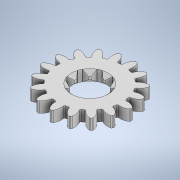
# Autodesk Inventor part: Gear_input
Saved by Autodesk Inventor 2020 (Build 240168000, 168)
## iProperties
Created: 2020-05-11
Part Number: Gear_input
Material: Generic
Document SubType Name: Modeling
Designer: avi41
Density: 1 g/cm^3
Appearance: Default
Author: avi41
Autodesk Inventor part; units mm, degrees
ref_plane "YZ Plane" through (0, 0, 0) normal (1, 0, 0) x (0, 1, 0)
ref_plane "XZ Plane" through (0, 0, 0) normal (0, 1, 0) x (-1, 0, 0)
ref_plane "XY Plane" through (0, 0, 0) normal (0, 0, 1) x (1, 0, 0)
sketch "Sketch1" plane through (0, 0, 0) normal (0, 1, 0) x (-1, 0, 0)
  arc A0 (0.3488, -8.9491) -> (-2.2796, -8.6609) centre (0, 0) ccw construction
  line L0 (0, -21.7523) -> (0, 17.3166) construction
  line L1 (-16.4294, 0) -> (16.4294, 0) construction
  arc A1 (0.3488, -8.9491) -> (-2.2796, -8.6609) centre (0, 0) ccw
  circle A2 centre (0, 0) radius 11.7353 construction
  circle A3 centre (0, 0) radius 10.5 construction
  line L2 (0, 0) -> (-4.0137, -11.0276) construction
  circle A4 centre (0, 0) radius 9.8668 construction
  line L3 (-3.3746, -9.2717) -> (5.3254, -12.4383) construction
  line L4 (3.5046, -9.8668) -> (-4.0266, -9.8668) construction
  arc A5 (-0.9533, -11.6965) -> (0.052, -9.2588) centre (-3.3746, -9.2717) ccw
  circle A6 centre (0, 0) radius 9.2647 construction
  arc A7 (0.3488, -8.9491) -> (0.052, -9.2588) centre (0.3609, -9.2577) ccw
  line L5 (-1.3339, -12.1661) -> (-0.7958, -7.2586) construction
  arc A8 (-2.057, -9.0276) -> (-1.6037, -11.6252) centre (1.2855, -9.7827) ccw
  arc A9 (-2.057, -9.0276) -> (-2.2796, -8.6609) centre (-2.3582, -8.9595) ccw
  line L6 (-0.9533, -11.6965) -> (-1.6037, -11.6252)
  point P0 (0, -9.8668)
  point P1 (-0.149, -9.2635)
  point P2 (0, -16.1711)
  point P3 (-0.1751, -10.4985)
  point P4 (-1.8617, -9.0757)
  point P5 (-3.504, -15.7869)
  point P6 (-0.1601, -15.8391)
  point P7 (-6.1857, -13.0529)
  point P8 (-5.7886, -14.7444)
  point P9 (-1.2807, -6.5842)
  dimension "d23" = 21
  dimension "d25" = 1.5441
  dimension "d26" = 1.2353
  dimension "d27" = 20
  dimension "d28" = 19.7336
  dimension "d29" = 20
  dimension "d30" = 0.3088
  dimension "d31" = 0.6177
  dimension "d32" = 0.9702
  constraints: 18 point on circle, 10 end point, 8 centre point, 7 coincident, 6 symmetric about line, 4 point on line, 3 tangent, 1 concentric, 1 horizontal, 8 other
  measures "d27" angle of L0 L2
  measures "d28" diameter of A4
  measures "d29" angle of L4 L3
  measures "d31" diameter of A7
  measures "d32" distance from line of point (-0.175, -10.499) L5
extrude "Extrusion1" add sketch "Sketch1" along normal mid plane 3
fillet "Fillet2" radius 0.4 2 edges at (0.9533, 0, -11.6965) (1.6037, 0, -11.6252)
pattern_circular "Circular Pattern2" count 17 over 360 about axis through (0, -10, 0) along (0, 1, 0) of "Extrusion1", "Fillet2"
sketch "Sketch3" plane through (0, 0, 0) normal (0, 1, 0) x (-1, 0, 0)
  line L0 (-7, 0) -> (7, 0) construction
  line L1 (0, 7) -> (0, -7) construction
  circle A0 centre (0, 0) radius 4.9 construction
  circle A1 centre (0, 0) radius 3.8 construction
  line L2 (-0.5, 4.8744) -> (-1.2405, 3.5918) construction
  line L3 (0.5, 4.8744) -> (1.2405, 3.5918) construction
  circle A2 centre (0, 0) radius 3.75 construction
  circle A3 centre (0, 0) radius 4.45 construction
  circle A4 centre (-1.3496, 3.7229) radius 0.16 construction
  circle A5 centre (1.3496, 3.7229) radius 0.16 construction
  circle A6 centre (0, 0) radius 3.8 construction
  line L4 (0.5, 4.8744) -> (1.2405, 3.5918) construction
  line L5 (-0.5, 4.8744) -> (-1.2405, 3.5918) construction
  arc A7 (-1.2951, 3.5725) -> (-1.211, 3.6429) centre (-1.3496, 3.7229) ccw construction
  arc A8 (1.211, 3.6429) -> (1.2951, 3.5725) centre (1.3496, 3.7229) ccw construction
  arc A9 (0.5, 4.8744) -> (-0.5, 4.8744) centre (0, 0) ccw construction
  circle A10 centre (0, 0) radius 3.8 construction
  circle A11 centre (0, 0) radius 3.8 construction
  circle A12 centre (0, 0) radius 4.45 construction
  circle A13 centre (0, 0) radius 3.75 construction
  circle A14 centre (0, 0) radius 4.9 construction
  arc A15 (-1.7196, 3.4323) -> (-1.6104, 3.4419) centre (-1.6782, 3.5868) ccw construction
  circle A16 centre (-1.6782, 3.5868) radius 0.16 construction
  arc A17 (-3.0932, 3.8003) -> (-3.8003, 3.0932) centre (0, 0) ccw construction
  line L6 (-3.0932, 3.8003) -> (-1.6626, 3.417) construction
  line L7 (-3.0932, 3.8003) -> (-1.6626, 3.417) construction
  line L8 (-3.8003, 3.0932) -> (-3.417, 1.6626) construction
  line L9 (-3.8003, 3.0932) -> (-3.417, 1.6626) construction
  arc A18 (-3.4419, 1.6104) -> (-3.4323, 1.7196) centre (-3.5868, 1.6782) ccw construction
  circle A19 centre (-3.5868, 1.6782) radius 0.16 construction
  circle A20 centre (0, 0) radius 3.8 construction
  circle A21 centre (0, 0) radius 3.8 construction
  circle A22 centre (0, 0) radius 4.45 construction
  circle A23 centre (0, 0) radius 3.75 construction
  circle A24 centre (0, 0) radius 4.9 construction
  arc A25 (-3.6429, 1.211) -> (-3.5725, 1.2951) centre (-3.7229, 1.3496) ccw construction
  circle A26 centre (-3.7229, 1.3496) radius 0.16 construction
  arc A27 (-4.8744, 0.5) -> (-4.8744, -0.5) centre (0, 0) ccw construction
  line L10 (-4.8744, 0.5) -> (-3.5918, 1.2405) construction
  line L11 (-4.8744, 0.5) -> (-3.5918, 1.2405) construction
  line L12 (-4.8744, -0.5) -> (-3.5918, -1.2405) construction
  line L13 (-4.8744, -0.5) -> (-3.5918, -1.2405) construction
  arc A28 (-3.5725, -1.2951) -> (-3.6429, -1.211) centre (-3.7229, -1.3496) ccw construction
  circle A29 centre (-3.7229, -1.3496) radius 0.16 construction
  circle A30 centre (0, 0) radius 3.8 construction
  circle A31 centre (0, 0) radius 3.8 construction
  circle A32 centre (0, 0) radius 4.45 construction
  circle A33 centre (0, 0) radius 3.75 construction
  circle A34 centre (0, 0) radius 4.9 construction
  arc A35 (-3.4323, -1.7196) -> (-3.4419, -1.6104) centre (-3.5868, -1.6782) ccw construction
  circle A36 centre (-3.5868, -1.6782) radius 0.16 construction
  arc A37 (-3.8003, -3.0932) -> (-3.0932, -3.8003) centre (0, 0) ccw construction
  line L14 (-3.8003, -3.0932) -> (-3.417, -1.6626) construction
  line L15 (-3.8003, -3.0932) -> (-3.417, -1.6626) construction
  line L16 (-3.0932, -3.8003) -> (-1.6626, -3.417) construction
  line L17 (-3.0932, -3.8003) -> (-1.6626, -3.417) construction
  arc A38 (-1.6104, -3.4419) -> (-1.7196, -3.4323) centre (-1.6782, -3.5868) ccw construction
  circle A39 centre (-1.6782, -3.5868) radius 0.16 construction
  circle A40 centre (0, 0) radius 3.8 construction
  circle A41 centre (0, 0) radius 3.8 construction
  circle A42 centre (0, 0) radius 4.45 construction
  circle A43 centre (0, 0) radius 3.75 construction
  circle A44 centre (0, 0) radius 4.9 construction
  arc A45 (-1.211, -3.6429) -> (-1.2951, -3.5725) centre (-1.3496, -3.7229) ccw construction
  circle A46 centre (-1.3496, -3.7229) radius 0.16 construction
  arc A47 (-0.5, -4.8744) -> (0.5, -4.8744) centre (0, 0) ccw construction
  line L18 (-0.5, -4.8744) -> (-1.2405, -3.5918) construction
  line L19 (-0.5, -4.8744) -> (-1.2405, -3.5918) construction
  line L20 (0.5, -4.8744) -> (1.2405, -3.5918) construction
  line L21 (0.5, -4.8744) -> (1.2405, -3.5918) construction
  arc A48 (1.2951, -3.5725) -> (1.211, -3.6429) centre (1.3496, -3.7229) ccw construction
  circle A49 centre (1.3496, -3.7229) radius 0.16 construction
  circle A50 centre (0, 0) radius 3.8 construction
  circle A51 centre (0, 0) radius 3.8 construction
  circle A52 centre (0, 0) radius 4.45 construction
  circle A53 centre (0, 0) radius 3.75 construction
  circle A54 centre (0, 0) radius 4.9 construction
  arc A55 (1.7196, -3.4323) -> (1.6104, -3.4419) centre (1.6782, -3.5868) ccw construction
  circle A56 centre (1.6782, -3.5868) radius 0.16 construction
  arc A57 (3.0932, -3.8003) -> (3.8003, -3.0932) centre (0, 0) ccw construction
  line L22 (3.0932, -3.8003) -> (1.6626, -3.417) construction
  line L23 (3.0932, -3.8003) -> (1.6626, -3.417) construction
  line L24 (3.8003, -3.0932) -> (3.417, -1.6626) construction
  line L25 (3.8003, -3.0932) -> (3.417, -1.6626) construction
  arc A58 (3.4419, -1.6104) -> (3.4323, -1.7196) centre (3.5868, -1.6782) ccw construction
  circle A59 centre (3.5868, -1.6782) radius 0.16 construction
  circle A60 centre (0, 0) radius 3.8 construction
  circle A61 centre (0, 0) radius 3.8 construction
  circle A62 centre (0, 0) radius 4.45 construction
  circle A63 centre (0, 0) radius 3.75 construction
  circle A64 centre (0, 0) radius 4.9 construction
  arc A65 (3.6429, -1.211) -> (3.5725, -1.2951) centre (3.7229, -1.3496) ccw construction
  circle A66 centre (3.7229, -1.3496) radius 0.16 construction
  arc A67 (4.8744, -0.5) -> (4.8744, 0.5) centre (0, 0) ccw construction
  line L26 (4.8744, -0.5) -> (3.5918, -1.2405) construction
  line L27 (4.8744, -0.5) -> (3.5918, -1.2405) construction
  line L28 (4.8744, 0.5) -> (3.5918, 1.2405) construction
  line L29 (4.8744, 0.5) -> (3.5918, 1.2405) construction
  arc A68 (3.5725, 1.2951) -> (3.6429, 1.211) centre (3.7229, 1.3496) ccw construction
  circle A69 centre (3.7229, 1.3496) radius 0.16 construction
  line L30 (0, -16.3542) -> (0, 16.3851) construction
  line L31 (-16.3961, 0) -> (16.2574, 0) construction
  circle A70 centre (0, 0) radius 4
  circle A71 centre (0, 0) radius 5.1 construction
  line L32 (1.4495, 4.8897) -> (0.2774, 3.9904) construction
  line L33 (-1.4495, 4.8897) -> (-0.2774, 3.9904) construction
  arc A72 (-1.3841, 4.8395) -> (-1.5295, 4.8652) centre (-1.4815, 4.7126) ccw
  arc A73 (1.5295, 4.8652) -> (1.3841, 4.8395) centre (1.4815, 4.7126) ccw
  line L34 (1.3841, 4.8395) -> (0.2774, 3.9904)
  line L35 (-1.3841, 4.8395) -> (-0.2774, 3.9904)
  circle A74 centre (0, 0) radius 5.1
  circle A75 centre (0, 0) radius 4.45 construction
  line L36 (-4.4825, 2.4326) -> (-3.0178, 2.6254) construction
  arc A76 (-4.4008, 2.4434) -> (-4.5218, 2.3587) centre (-4.3799, 2.2847) ccw
  line L37 (-2.4434, 4.4008) -> (-2.6254, 3.0178)
  arc A77 (-2.3587, 4.5218) -> (-2.4434, 4.4008) centre (-2.2847, 4.3799) ccw
  line L38 (-2.4326, 4.4825) -> (-2.6254, 3.0178) construction
  line L39 (-4.4008, 2.4434) -> (-3.0178, 2.6254)
  line L40 (-4.8897, -1.4495) -> (-3.9904, -0.2774) construction
  arc A78 (-4.8395, -1.3841) -> (-4.8652, -1.5295) centre (-4.7126, -1.4815) ccw
  line L41 (-4.8395, 1.3841) -> (-3.9904, 0.2774)
  arc A79 (-4.8652, 1.5295) -> (-4.8395, 1.3841) centre (-4.7126, 1.4815) ccw
  line L42 (-4.8897, 1.4495) -> (-3.9904, 0.2774) construction
  line L43 (-4.8395, -1.3841) -> (-3.9904, -0.2774)
  line L44 (-2.4326, -4.4825) -> (-2.6254, -3.0178) construction
  arc A80 (-2.4434, -4.4008) -> (-2.3587, -4.5218) centre (-2.2847, -4.3799) ccw
  line L45 (-4.4008, -2.4434) -> (-3.0178, -2.6254)
  arc A81 (-4.5218, -2.3587) -> (-4.4008, -2.4434) centre (-4.3799, -2.2847) ccw
  line L46 (-4.4825, -2.4326) -> (-3.0178, -2.6254) construction
  line L47 (-2.4434, -4.4008) -> (-2.6254, -3.0178)
  line L48 (1.4495, -4.8897) -> (0.2774, -3.9904) construction
  arc A82 (1.3841, -4.8395) -> (1.5295, -4.8652) centre (1.4815, -4.7126) ccw
  line L49 (-1.3841, -4.8395) -> (-0.2774, -3.9904)
  arc A83 (-1.5295, -4.8652) -> (-1.3841, -4.8395) centre (-1.4815, -4.7126) ccw
  line L50 (-1.4495, -4.8897) -> (-0.2774, -3.9904) construction
  line L51 (1.3841, -4.8395) -> (0.2774, -3.9904)
  line L52 (4.4825, -2.4326) -> (3.0178, -2.6254) construction
  arc A84 (4.4008, -2.4434) -> (4.5218, -2.3587) centre (4.3799, -2.2847) ccw
  line L53 (2.4434, -4.4008) -> (2.6254, -3.0178)
  arc A85 (2.3587, -4.5218) -> (2.4434, -4.4008) centre (2.2847, -4.3799) ccw
  line L54 (2.4326, -4.4825) -> (2.6254, -3.0178) construction
  line L55 (4.4008, -2.4434) -> (3.0178, -2.6254)
  line L56 (4.8897, 1.4495) -> (3.9904, 0.2774) construction
  arc A86 (4.8395, 1.3841) -> (4.8652, 1.5295) centre (4.7126, 1.4815) ccw
  line L57 (4.8395, -1.3841) -> (3.9904, -0.2774)
  arc A87 (4.8652, -1.5295) -> (4.8395, -1.3841) centre (4.7126, -1.4815) ccw
  line L58 (4.8897, -1.4495) -> (3.9904, -0.2774) construction
  line L59 (4.8395, 1.3841) -> (3.9904, 0.2774)
  circle A88 centre (0, 0) radius 3.8 construction
  circle A89 centre (0, 0) radius 3.8 construction
  circle A90 centre (0, 0) radius 4.45 construction
  circle A91 centre (0, 0) radius 3.75 construction
  circle A92 centre (0, 0) radius 4.9 construction
  arc A93 (3.4323, 1.7196) -> (3.4419, 1.6104) centre (3.5868, 1.6782) ccw construction
  circle A94 centre (3.5868, 1.6782) radius 0.16 construction
  arc A95 (3.8003, 3.0932) -> (3.0932, 3.8003) centre (0, 0) ccw construction
  line L60 (3.8003, 3.0932) -> (3.417, 1.6626) construction
  line L61 (3.8003, 3.0932) -> (3.417, 1.6626) construction
  line L62 (3.0932, 3.8003) -> (1.6626, 3.417) construction
  line L63 (3.0932, 3.8003) -> (1.6626, 3.417) construction
  arc A96 (1.6104, 3.4419) -> (1.7196, 3.4323) centre (1.6782, 3.5868) ccw construction
  circle A97 centre (1.6782, 3.5868) radius 0.16 construction
  line L64 (2.4326, 4.4825) -> (2.6254, 3.0178) construction
  arc A98 (2.4434, 4.4008) -> (2.3587, 4.5218) centre (2.2847, 4.3799) ccw
  line L65 (4.4008, 2.4434) -> (3.0178, 2.6254)
  arc A99 (4.5218, 2.3587) -> (4.4008, 2.4434) centre (4.3799, 2.2847) ccw
  line L66 (4.4825, 2.4326) -> (3.0178, 2.6254) construction
  line L67 (2.4434, 4.4008) -> (2.6254, 3.0178)
  point P0 (-0.7854, 4.3801)
  point P1 (0.7854, 4.3801)
  point P2 (-3.6526, 2.5419)
  point P3 (-2.5419, 3.6526)
  point P4 (-4.3801, -0.7854)
  point P5 (-4.3801, 0.7854)
  point P6 (-2.5419, -3.6526)
  point P7 (-3.6526, -2.5419)
  point P8 (0.7854, -4.3801)
  point P9 (-0.7854, -4.3801)
  point P10 (3.6526, -2.5419)
  point P11 (2.5419, -3.6526)
  point P12 (4.3801, 0.7854)
  point P13 (4.3801, -0.7854)
  point P14 (1.3297, 2.7449)
  point P15 (2.9719, 0.6856)
  point P16 (2.9751, 0.6718)
  point P17 (2.389, -1.8961)
  point P18 (2.3802, -1.9072)
  point P19 (0.0071, -3.05)
  point P20 (-0.0071, -3.05)
  point P21 (-2.3802, -1.9072)
  point P22 (-2.389, -1.8961)
  point P23 (-2.9751, 0.6718)
  point P24 (-2.9719, 0.6856)
  point P25 (-1.3297, 2.7449)
  point P26 (0.7854, 4.3801)
  point P27 (-0.7854, 4.3801)
  point P28 (-2.5419, 3.6526)
  point P29 (-3.6526, 2.5419)
  point P30 (-4.3801, 0.7854)
  point P31 (-4.3801, -0.7854)
  point P32 (-3.6526, -2.5419)
  point P33 (-2.5419, -3.6526)
  point P34 (-0.7854, -4.3801)
  point P35 (0.7854, -4.3801)
  point P36 (2.5419, -3.6526)
  point P37 (3.6526, -2.5419)
  point P38 (4.3801, -0.7854)
  point P39 (4.3801, 0.7854)
  point P40 (3.9904, 0.2774)
  point P41 (4.8652, 1.5295)
  point P42 (-2.3587, 4.5218)
  point P43 (-2.6254, 3.0178)
  point P44 (-3.0178, 2.6254)
  point P45 (-4.5218, 2.3587)
  point P46 (-4.8652, 1.5295)
  point P47 (-3.9904, 0.2774)
  point P48 (-3.9904, -0.2774)
  point P49 (-4.8652, -1.5295)
  point P50 (-4.5218, -2.3587)
  point P51 (-3.0178, -2.6254)
  point P52 (-2.6254, -3.0178)
  point P53 (-2.3587, -4.5218)
  point P54 (-1.5295, -4.8652)
  point P55 (-0.2774, -3.9904)
  point P56 (0.2774, -3.9904)
  point P57 (1.5295, -4.8652)
  point P58 (2.3587, -4.5218)
  point P59 (2.6254, -3.0178)
  point P60 (3.0178, -2.6254)
  point P61 (4.5218, -2.3587)
  point P62 (4.8652, -1.5295)
  point P63 (3.9904, -0.2774)
  point P64 (2.5419, 3.6526)
  point P65 (3.6526, 2.5419)
  point P66 (3.6526, 2.5419)
  point P67 (2.5419, 3.6526)
  point P68 (2.6254, 3.0178)
  point P69 (2.3587, 4.5218)
  point P70 (4.5218, 2.3587)
  point P71 (3.0178, 2.6254)
  dimension "d36" = 9.8
  dimension "d37" = 7.6
  dimension "d38" = 30
  dimension "d39" = 7.5
  dimension "d40" = 0.65
  dimension "d41" = 1.5708
  dimension "d42" = 0.32
  dimension "d43" = 360
  dimension "d58" = 8
  dimension "d59" = 10.2
  dimension "d60" = 8.9
  dimension "d61" = 1.5708
  dimension "d68" = 360
  dimension "d74" = 60
  constraints: 152 point on circle, 132 end point, 100 centre point, 64 point on line, 61 coincident, 8 tangent, 6 equal radius, 3 collinear, 3 midpoint, 2 horizontal, 2 vertical, 1 symmetric about line, 465 other
  measures "d36" diameter of A0
  measures "d37" diameter of A1
  measures "d38" angle of L1 L2
  measures "d39" diameter of A2
  measures "d40" radial gap between concentric circles of A3 A1
  measures "d41" distance of A3.end A3.start
  measures "d42" diameter of A4
  measures "d58" diameter of A70
  measures "d59" diameter of A71
  measures "d60" diameter of A75
  measures "d61" distance of A75.start A75.end
  measures "d74" angle of L64 L34
extrude "Extrusion4" cut sketch "Sketch3" against normal through all both and the other way through all contours A70 | A70 L65 A99 A74 A86 L59 | L57 A87 A74 A84 L55 A70 | A70 L34 A73 A74 A98 L67 | L53 A85 A74 A82 L51 A70 | A70 L37 A77 A74 A72 L35 | L49 A83 A74 A80 L47 A70 | A70 L41 A79 A74 A76 L39 | L45 A81 A74 A78 L43 A70
sketch "Sketch4" plane through (0, 1.5, 0) normal (0, 1, 0) x (1, 0, 0)
  circle A0 centre (0, 0) radius 5.1
  arc A1 (-2.4434, -4.4008) -> (-2.3587, -4.5218) centre (-2.2847, -4.3799) ccw projected
  line L0 (-2.4434, -4.4008) -> (-2.6254, -3.0178) projected
  arc A2 (-3.0178, -2.6254) -> (-2.6254, -3.0178) centre (0, 0) ccw projected
  line L1 (-3.0178, -2.6254) -> (-4.4008, -2.4434) projected
  arc A3 (-4.5218, -2.3587) -> (-4.4008, -2.4434) centre (-4.3799, -2.2847) ccw projected
  arc A4 (-4.8652, -1.5295) -> (-4.5218, -2.3587) centre (0, 0) ccw projected
  arc A5 (-4.8395, -1.3841) -> (-4.8652, -1.5295) centre (-4.7126, -1.4815) ccw projected
  line L2 (-4.8395, -1.3841) -> (-3.9904, -0.2774) projected
  arc A6 (-3.9904, 0.2774) -> (-3.9904, -0.2774) centre (0, 0) ccw projected
  line L3 (-3.9904, 0.2774) -> (-4.8395, 1.3841) projected
  arc A7 (-4.8652, 1.5295) -> (-4.8395, 1.3841) centre (-4.7126, 1.4815) ccw projected
  arc A8 (-4.5218, 2.3587) -> (-4.8652, 1.5295) centre (0, 0) ccw projected
  arc A9 (-4.4008, 2.4434) -> (-4.5218, 2.3587) centre (-4.3799, 2.2847) ccw projected
  line L4 (-4.4008, 2.4434) -> (-3.0178, 2.6254) projected
  arc A10 (-2.6254, 3.0178) -> (-3.0178, 2.6254) centre (0, 0) ccw projected
  line L5 (-2.6254, 3.0178) -> (-2.4434, 4.4008) projected
  arc A11 (-2.3587, 4.5218) -> (-2.4434, 4.4008) centre (-2.2847, 4.3799) ccw projected
  arc A12 (-1.5295, 4.8652) -> (-2.3587, 4.5218) centre (0, 0) ccw projected
  arc A13 (-1.3841, 4.8395) -> (-1.5295, 4.8652) centre (-1.4815, 4.7126) ccw projected
  line L6 (-1.3841, 4.8395) -> (-0.2774, 3.9904) projected
  arc A14 (0.2774, 3.9904) -> (-0.2774, 3.9904) centre (0, 0) ccw projected
  line L7 (0.2774, 3.9904) -> (1.3841, 4.8395) projected
  arc A15 (1.5295, 4.8652) -> (1.3841, 4.8395) centre (1.4815, 4.7126) ccw projected
  arc A16 (2.3587, 4.5218) -> (1.5295, 4.8652) centre (0, 0) ccw projected
  arc A17 (2.4434, 4.4008) -> (2.3587, 4.5218) centre (2.2847, 4.3799) ccw projected
  line L8 (2.4434, 4.4008) -> (2.6254, 3.0178) projected
  arc A18 (3.0178, 2.6254) -> (2.6254, 3.0178) centre (0, 0) ccw projected
  line L9 (3.0178, 2.6254) -> (4.4008, 2.4434) projected
  arc A19 (4.5218, 2.3587) -> (4.4008, 2.4434) centre (4.3799, 2.2847) ccw projected
  arc A20 (4.8652, 1.5295) -> (4.5218, 2.3587) centre (0, 0) ccw projected
  arc A21 (4.8395, 1.3841) -> (4.8652, 1.5295) centre (4.7126, 1.4815) ccw projected
  line L10 (4.8395, 1.3841) -> (3.9904, 0.2774) projected
  arc A22 (3.9904, -0.2774) -> (3.9904, 0.2774) centre (0, 0) ccw projected
  line L11 (3.9904, -0.2774) -> (4.8395, -1.3841) projected
  arc A23 (4.8652, -1.5295) -> (4.8395, -1.3841) centre (4.7126, -1.4815) ccw projected
  arc A24 (4.5218, -2.3587) -> (4.8652, -1.5295) centre (0, 0) ccw projected
  arc A25 (4.4008, -2.4434) -> (4.5218, -2.3587) centre (4.3799, -2.2847) ccw projected
  line L12 (4.4008, -2.4434) -> (3.0178, -2.6254) projected
  arc A26 (2.6254, -3.0178) -> (3.0178, -2.6254) centre (0, 0) ccw projected
  line L13 (2.6254, -3.0178) -> (2.4434, -4.4008) projected
  arc A27 (2.3587, -4.5218) -> (2.4434, -4.4008) centre (2.2847, -4.3799) ccw projected
  arc A28 (1.5295, -4.8652) -> (2.3587, -4.5218) centre (0, 0) ccw projected
  arc A29 (1.3841, -4.8395) -> (1.5295, -4.8652) centre (1.4815, -4.7126) ccw projected
  line L14 (1.3841, -4.8395) -> (0.2774, -3.9904) projected
  arc A30 (-0.2774, -3.9904) -> (0.2774, -3.9904) centre (0, 0) ccw projected
  line L15 (-0.2774, -3.9904) -> (-1.3841, -4.8395) projected
  arc A31 (-1.5295, -4.8652) -> (-1.3841, -4.8395) centre (-1.4815, -4.7126) ccw projected
  arc A32 (-2.3587, -4.5218) -> (-1.5295, -4.8652) centre (0, 0) ccw projected
  arc A33 (2.057, 9.0276) -> (2.2796, 8.6609) centre (2.3582, 8.9595) ccw projected
  arc A34 (2.057, 9.0276) -> (1.7121, 11.4431) centre (-1.2855, 9.7827) ccw projected
  arc A35 (1.7121, 11.4431) -> (1.4058, 11.6469) centre (1.3622, 11.2493) ccw projected
  line L16 (1.4058, 11.6469) -> (1.1513, 11.6748) projected
  arc A36 (1.1513, 11.6748) -> (0.8081, 11.5422) centre (1.1077, 11.2772) ccw projected
  arc A37 (0.8081, 11.5422) -> (-0.052, 9.2588) centre (3.3746, 9.2717) ccw projected
  arc A38 (-0.3488, 8.9491) -> (-0.052, 9.2588) centre (-0.3609, 9.2577) ccw projected
  arc A39 (-0.3488, 8.9491) -> (-1.003, 8.8995) centre (0, 0) ccw projected
  arc A40 (-1.343, 9.1611) -> (-1.003, 8.8995) centre (-1.0376, 9.2064) ccw projected
  arc A41 (-1.343, 9.1611) -> (-2.5373, 11.2889) centre (-4.7326, 8.6577) ccw projected
  arc A42 (-2.5373, 11.2889) -> (-2.8965, 11.3682) centre (-2.7935, 10.9817) ccw projected
  line L17 (-2.8965, 11.3682) -> (-3.1439, 11.3023) projected
  arc A43 (-3.1439, 11.3023) -> (-3.416, 11.0547) centre (-3.0409, 10.9158) ccw projected
  arc A44 (-3.416, 11.0547) -> (-3.3932, 8.6148) centre (-0.2026, 9.8647) ccw projected
  arc A45 (-3.5581, 8.2188) -> (-3.3932, 8.6148) centre (-3.6807, 8.5022) ccw projected
  arc A46 (-3.5581, 8.2188) -> (-4.1501, 7.9363) centre (0, 0) ccw projected
  arc A47 (-4.5617, 8.0573) -> (-4.1501, 7.9363) centre (-4.2932, 8.2099) ccw projected
  arc A48 (-4.5617, 8.0573) -> (-6.4439, 9.61) centre (-7.5405, 6.3635) ccw projected
  arc A49 (-6.4439, 9.61) -> (-6.8076, 9.5542) centre (-6.5719, 9.231) ccw projected
  line L18 (-6.8076, 9.5542) -> (-7.0145, 9.4034) projected
  arc A50 (-7.0145, 9.4034) -> (-7.1788, 9.0742) centre (-6.7788, 9.0802) ccw projected
  arc A51 (-7.1788, 9.0742) -> (-6.2761, 6.8073) centre (-3.7524, 9.1254) ccw projected
  arc A52 (-6.2867, 6.3785) -> (-6.2761, 6.8073) centre (-6.5035, 6.5984) ccw projected
  arc A53 (-6.2867, 6.3785) -> (-6.7368, 5.9011) centre (0, 0) ccw projected
  arc A54 (-7.1643, 5.8653) -> (-6.7368, 5.9011) centre (-6.9691, 6.1046) ccw projected
  arc A55 (-7.1643, 5.8653) -> (-9.4803, 6.6332) centre (-9.3301, 3.2098) ccw projected
  arc A56 (-9.4803, 6.6332) -> (-9.7993, 6.4499) centre (-9.4628, 6.2336) ccw projected
  line L19 (-9.7993, 6.4499) -> (-9.9377, 6.2345) projected
  arc A57 (-9.9377, 6.2345) -> (-9.972, 5.8682) centre (-9.6012, 6.0182) ccw projected
  arc A58 (-9.972, 5.8682) -> (-8.3114, 4.0804) centre (-6.7955, 7.1536) ccw projected
  arc A59 (-8.1664, 3.6767) -> (-8.3114, 4.0804) centre (-8.448, 3.8035) ccw projected
  arc A60 (-8.1664, 3.6767) -> (-8.4136, 3.069) centre (0, 0) ccw projected
  arc A61 (-8.7993, 2.8812) -> (-8.4136, 3.069) centre (-8.7037, 3.1749) ccw projected
  arc A62 (-8.7993, 2.8812) -> (-11.2363, 2.7606) centre (-9.8596, -0.3773) ccw projected
  arc A63 (-11.2363, 2.7606) -> (-11.4675, 2.4744) centre (-11.0756, 2.3943) ccw projected
  line L20 (-11.4675, 2.4744) -> (-11.5188, 2.2236) projected
  arc A64 (-11.5188, 2.2236) -> (-11.4184, 1.8696) centre (-11.1269, 2.1435) ccw projected
  arc A65 (-11.4184, 1.8696) -> (-9.2241, 0.8025) centre (-8.9208, 4.2157) ccw projected
  arc A66 (-8.9431, 0.4784) -> (-9.2241, 0.8025) centre (-9.2515, 0.4949) ccw projected
  arc A67 (-8.9431, 0.4784) -> (-8.9541, -0.1776) centre (0, 0) ccw projected
  arc A68 (-9.2459, -0.492) -> (-8.9541, -0.1776) centre (-9.2629, -0.1837) ccw projected
  arc A69 (-9.2459, -0.492) -> (-11.4748, -1.4848) centre (-9.0575, -3.9135) ccw projected
  arc A70 (-11.4748, -1.4848) -> (-11.587, -1.8352) centre (-11.1926, -1.7683) ccw projected
  line L21 (-11.587, -1.8352) -> (-11.5442, -2.0876) projected
  arc A71 (-11.5442, -2.0876) -> (-11.3228, -2.3814) centre (-11.1498, -2.0207) ccw projected
  arc A72 (-11.3228, -2.3814) -> (-8.8911, -2.5838) centre (-9.8413, 0.7085) ccw projected
  arc A73 (-8.512, -2.7845) -> (-8.8911, -2.5838) centre (-8.8055, -2.8806) ccw projected
  arc A74 (-8.512, -2.7845) -> (-8.2853, -3.4002) centre (0, 0) ccw projected
  arc A75 (-8.4438, -3.7988) -> (-8.2853, -3.4002) centre (-8.571, -3.5174) ccw projected
  arc A76 (-8.4438, -3.7988) -> (-10.1636, -5.5297) centre (-7.0321, -6.9212) ccw projected
  arc A77 (-10.1636, -5.5297) -> (-10.1416, -5.897) centre (-9.798, -5.6922) ccw projected
  line L22 (-10.1416, -5.897) -> (-10.0105, -6.1169) projected
  arc A78 (-10.0105, -6.1169) -> (-9.6979, -6.3109) centre (-9.6669, -5.9121) ccw projected
  arc A79 (-9.6979, -6.3109) -> (-7.3574, -5.6212) centre (-9.4327, -2.8945) ccw projected
  arc A80 (-6.9313, -5.6714) -> (-7.3574, -5.6212) centre (-7.1703, -5.867) ccw projected
  arc A81 (-6.9313, -5.6714) -> (-6.4976, -6.1636) centre (0, 0) ccw projected
  arc A82 (-6.5013, -6.5925) -> (-6.4976, -6.1636) centre (-6.7216, -6.3761) ccw projected
  arc A83 (-6.5013, -6.5925) -> (-7.4797, -8.8278) centre (-4.057, -8.9941) ccw projected
  arc A84 (-7.4797, -8.8278) -> (-7.3265, -9.1624) centre (-7.0801, -8.8472) ccw projected
  line L23 (-7.3265, -9.1624) -> (-7.1248, -9.32) projected
  arc A85 (-7.1248, -9.32) -> (-6.7633, -9.388) centre (-6.8785, -9.0049) ccw projected
  arc A86 (-6.7633, -9.388) -> (-4.8299, -7.8994) centre (-7.7501, -6.1065) ccw projected
  arc A87 (-4.4145, -7.7923) -> (-4.8299, -7.8994) centre (-4.5667, -8.061) ccw projected
  arc A88 (-4.4145, -7.7923) -> (-3.8323, -8.0945) centre (0, 0) ccw projected
  arc A89 (-3.6808, -8.4959) -> (-3.8323, -8.0945) centre (-3.9644, -8.3737) ccw projected
  arc A90 (-3.6808, -8.4959) -> (-3.7856, -10.9337) centre (-0.534, -9.8523) ccw projected
  arc A91 (-3.7856, -10.9337) -> (-3.5219, -11.1903) centre (-3.406, -10.8074) ccw projected
  line L24 (-3.5219, -11.1903) -> (-3.2769, -11.2645) projected
  arc A92 (-3.2769, -11.2645) -> (-2.9152, -11.1972) centre (-3.161, -10.8816) ccw projected
  arc A93 (-2.9152, -11.1972) -> (-1.6502, -9.1107) centre (-5.0209, -8.4938) ccw projected
  arc A94 (-1.3015, -8.8608) -> (-1.6502, -9.1107) centre (-1.3464, -9.1664) ccw projected
  arc A95 (-1.3015, -8.8608) -> (-0.6494, -8.9323) centre (0, 0) ccw projected
  arc A96 (-0.3632, -9.2519) -> (-0.6494, -8.9323) centre (-0.6718, -9.2403) ccw projected
  arc A97 (-0.3632, -9.2519) -> (0.4197, -11.5629) centre (3.0611, -9.3799) ccw projected
  arc A98 (0.4197, -11.5629) -> (0.7583, -11.7069) centre (0.7281, -11.308) ccw projected
  line L25 (0.7583, -11.7069) -> (1.0136, -11.6876) projected
  arc A99 (1.0136, -11.6876) -> (1.3265, -11.4942) centre (0.9833, -11.2887) ccw projected
  arc A100 (1.3265, -11.4942) -> (1.7525, -9.0916) centre (-1.6135, -9.734) ccw projected
  arc A101 (1.9873, -8.7326) -> (1.7525, -9.0916) centre (2.0558, -9.0337) ccw projected
  arc A102 (1.9873, -8.7326) -> (2.6212, -8.5637) centre (0, 0) ccw projected
  arc A103 (3.0035, -8.7583) -> (2.6212, -8.5637) centre (2.7116, -8.859) ccw projected
  arc A104 (3.0035, -8.7583) -> (4.5684, -10.6304) centre (6.2428, -7.6407) ccw projected
  arc A105 (4.5684, -10.6304) -> (4.9361, -10.6424) centre (4.7638, -10.2814) ccw projected
  line L26 (4.9361, -10.6424) -> (5.1671, -10.5322) projected
  arc A106 (5.1671, -10.5322) -> (5.3891, -10.2388) centre (4.9949, -10.1712) ccw projected
  arc A107 (5.3891, -10.2388) -> (4.9184, -7.8446) centre (2.0118, -9.6595) ccw projected
  arc A108 (5.0077, -7.425) -> (4.9184, -7.8446) centre (5.1803, -7.6811) ccw projected
  arc A109 (5.0077, -7.425) -> (5.5378, -7.0385) centre (0, 0) ccw projected
  arc A110 (5.9646, -7.0819) -> (5.5378, -7.0385) centre (5.7287, -7.2813) ccw projected
  arc A111 (5.9646, -7.0819) -> (8.1, -8.2623) centre (8.5814, -4.8696) ccw projected
  arc A112 (8.1, -8.2623) -> (8.4473, -8.1407) centre (8.1562, -7.8662) ccw projected
  line L27 (8.4473, -8.1407) -> (8.6229, -7.9544) projected
  arc A113 (8.6229, -7.9544) -> (8.7239, -7.6006) centre (8.3319, -7.68) ccw projected
  arc A114 (8.7239, -7.6006) -> (7.4201, -5.5382) centre (5.3653, -8.2805) ccw projected
  arc A115 (7.3517, -5.1147) -> (7.4201, -5.5382) centre (7.6052, -5.291) ccw projected
  arc A116 (7.3517, -5.1147) -> (7.7064, -4.5628) centre (0, 0) ccw projected
  arc A117 (8.12, -4.449) -> (7.7064, -4.5628) centre (7.9722, -4.7201) ccw projected
  arc A118 (8.12, -4.449) -> (10.5377, -4.7783) centre (9.761, -1.4408) ccw projected
  arc A119 (10.5377, -4.7783) -> (10.8176, -4.5394) centre (10.4471, -4.3887) ccw projected
  line L28 (10.8176, -4.5394) -> (10.9141, -4.3023) projected
  arc A120 (10.9141, -4.3023) -> (10.8805, -3.9359) centre (10.5436, -4.1516) ccw projected
  arc A121 (10.8805, -3.9359) -> (8.9196, -2.4838) centre (7.9943, -5.7831) ccw projected
  arc A122 (8.7029, -2.1135) -> (8.9196, -2.4838) centre (9.003, -2.1864) ccw projected
  arc A123 (8.7029, -2.1135) -> (8.8343, -1.4708) centre (0, 0) ccw projected
  arc A124 (9.1789, -1.2153) -> (8.8343, -1.4708) centre (9.1389, -1.5215) ccw projected
  arc A125 (9.1789, -1.2153) -> (11.5523, -0.6489) centre (9.6223, 2.1826) ccw projected
  arc A126 (11.5523, -0.6489) -> (11.7269, -0.3251) centre (11.327, -0.3184) ccw projected
  line L29 (11.7269, -0.3251) -> (11.7312, -0.0692) projected
  arc A127 (11.7312, -0.0692) -> (11.5675, 0.2603) centre (11.3313, -0.0624) ccw projected
  arc A128 (11.5675, 0.2603) -> (9.2145, 0.9061) centre (9.5436, -2.5048) ccw projected
  arc A129 (8.8787, 1.1731) -> (9.2145, 0.9061) centre (9.1849, 1.2135) ccw projected
  arc A130 (8.8787, 1.1731) -> (8.769, 1.8198) centre (0, 0) ccw projected
  arc A131 (8.9981, 2.1826) -> (8.769, 1.8198) centre (9.0714, 1.8826) ccw projected
  arc A132 (8.9981, 2.1826) -> (11.0066, 3.568) centre (8.1841, 5.5112) ccw projected
  arc A133 (11.0066, 3.568) -> (11.0525, 3.9331) centre (10.6771, 3.7949) ccw projected
  line L30 (11.0525, 3.9331) -> (10.964, 4.1733) projected
  arc A134 (10.964, 4.1733) -> (10.6924, 4.4214) centre (10.5887, 4.0351) ccw projected
  arc A135 (10.6924, 4.4214) -> (8.265, 4.1736) centre (9.8039, 1.1119) ccw projected
  arc A136 (7.8554, 4.3012) -> (8.265, 4.1736) centre (8.1263, 4.4495) ccw projected
  arc A137 (7.8554, 4.3012) -> (7.5195, 4.8647) centre (0, 0) ccw projected
  arc A138 (7.602, 5.2857) -> (7.5195, 4.8647) centre (7.7788, 5.0324) ccw projected
  arc A139 (7.602, 5.2857) -> (8.9744, 7.3031) centre (5.6406, 8.0955) ccw projected
  arc A140 (8.9744, 7.3031) -> (8.8853, 7.6601) centre (8.5853, 7.3956) ccw projected
  line L31 (8.8853, 7.6601) -> (8.7161, 7.8522) projected
  arc A141 (8.7161, 7.8522) -> (8.3731, 7.9854) centre (8.416, 7.5877) ccw projected
  arc A142 (8.3731, 7.9854) -> (6.1992, 6.8774) centre (8.7402, 4.5784) ccw projected
  arc A143 (5.7712, 6.8485) -> (6.1992, 6.8774) centre (5.9702, 7.0846) ccw projected
  arc A144 (5.7712, 6.8485) -> (5.2544, 7.2525) centre (0, 0) ccw projected
  arc A145 (5.1793, 7.6749) -> (5.2544, 7.2525) centre (5.4356, 7.5026) ccw projected
  arc A146 (5.1793, 7.6749) -> (5.7302, 10.0519) centre (2.3353, 9.5864) ccw projected
  arc A147 (5.7302, 10.0519) -> (5.5182, 10.3526) centre (5.3339, 9.9976) ccw projected
  line L32 (5.5182, 10.3526) -> (5.291, 10.4705) projected
  arc A148 (5.291, 10.4705) -> (4.9231, 10.4709) centre (5.1067, 10.1155) ccw projected
  arc A149 (4.9231, 10.4709) -> (3.2962, 8.6524) centre (6.4961, 7.4266) ccw projected
  arc A150 (2.9075, 8.4708) -> (3.2962, 8.6524) centre (3.0078, 8.7629) ccw projected
  arc A151 (2.9075, 8.4708) -> (2.2796, 8.6609) centre (0, 0) ccw projected
  constraints: 1 centre point, 1 coincident, 1 concentric
extrude "Extrusion5" [suppressed]
mirror "Mirror1" [suppressed]
chamfer "Chamfer1" [suppressed]
chamfer "Chamfer2" [suppressed]
sketch "Sketch6" plane through (0, 0, 0) normal (0, 0, 1) x (1, 0, 0)
  line L0 (-4.5218, 1.5) -> (-4.8652, 1.5) projected
  line L1 (-4.5218, -1.5) -> (-4.5218, 1.5) projected
  line L2 (-4.8652, -1.5) -> (-4.5218, -1.5) projected
  line L3 (-4.8652, -1.5) -> (-4.8652, 1.5) projected
  line L4 (0, 2.1) -> (0, -2.1) projected
  line L5 (-2.4434, -1.5) -> (-2.3587, -1.5) projected
  line L6 (-2.3587, -1.5) -> (-1.5295, -1.5) projected
  line L7 (-1.5295, -1.5) -> (-1.3841, -1.5) projected
  line L8 (-1.3841, -1.5) -> (-0.2774, -1.5) projected
  line L9 (-0.2774, -1.5) -> (0.2774, -1.5) projected
  line L10 (0.2774, -1.5) -> (1.3841, -1.5) projected
  line L11 (1.3841, -1.5) -> (1.5295, -1.5) projected
  line L12 (1.5295, -1.5) -> (2.3587, -1.5) projected
  line L13 (2.3587, -1.5) -> (2.4434, -1.5) projected
  line L14 (2.4434, -1.5) -> (2.6254, -1.5) projected
  line L15 (2.6254, -1.5) -> (3.0178, -1.5) projected
  line L16 (3.0178, -1.5) -> (4.4008, -1.5) projected
  line L17 (4.4008, -1.5) -> (4.5218, -1.5) projected
  line L18 (4.5218, -1.5) -> (4.8652, -1.5) projected
  line L19 (4.8652, -1.5) -> (4.8395, -1.5) projected
  line L20 (4.8395, -1.5) -> (3.9904, -1.5) projected
  line L21 (3.9904, -1.5) -> (3.9904, -1.5) projected
  line L22 (3.9904, -1.5) -> (4.8395, -1.5) projected
  line L23 (4.8395, -1.5) -> (4.8652, -1.5) projected
  line L24 (4.8652, -1.5) -> (4.5218, -1.5) projected
  line L25 (4.5218, -1.5) -> (4.4008, -1.5) projected
  line L26 (4.4008, -1.5) -> (3.0178, -1.5) projected
  line L27 (3.0178, -1.5) -> (2.6254, -1.5) projected
  line L28 (2.6254, -1.5) -> (2.4434, -1.5) projected
  line L29 (2.4434, -1.5) -> (2.3587, -1.5) projected
  line L30 (2.3587, -1.5) -> (1.5295, -1.5) projected
  line L31 (1.5295, -1.5) -> (1.3841, -1.5) projected
  line L32 (1.3841, -1.5) -> (0.2774, -1.5) projected
  line L33 (0.2774, -1.5) -> (-0.2774, -1.5) projected
  line L34 (-0.2774, -1.5) -> (-1.3841, -1.5) projected
  line L35 (-1.3841, -1.5) -> (-1.5295, -1.5) projected
  line L36 (-1.5295, -1.5) -> (-2.3587, -1.5) projected
  line L37 (-2.3587, -1.5) -> (-2.4434, -1.5) projected
  line L38 (-2.4434, -1.5) -> (-2.6254, -1.5) projected
  line L39 (-2.6254, -1.5) -> (-3.0178, -1.5) projected
  line L40 (-3.0178, -1.5) -> (-4.4008, -1.5) projected
  line L41 (-4.4008, -1.5) -> (-4.5218, -1.5) projected
  line L42 (-4.5218, -1.5) -> (-4.8652, -1.5) projected
  line L43 (-4.8652, -1.5) -> (-4.8395, -1.5) projected
  line L44 (-4.8395, -1.5) -> (-3.9904, -1.5) projected
  line L45 (-3.9904, -1.5) -> (-3.9904, -1.5) projected
  line L46 (-3.9904, -1.5) -> (-4.8395, -1.5) projected
  line L47 (-4.8395, -1.5) -> (-4.8652, -1.5) projected
  line L48 (-4.8652, -1.5) -> (-4.5218, -1.5) projected
  line L49 (-4.5218, -1.5) -> (-4.4008, -1.5) projected
  line L50 (-4.4008, -1.5) -> (-3.0178, -1.5) projected
  line L51 (-3.0178, -1.5) -> (-2.6254, -1.5) projected
  line L52 (-2.6254, -1.5) -> (-2.4434, -1.5) projected
  line L53 (-0.3488, -1.5) -> (-0.052, -1.5) projected
  line L54 (-0.052, -1.5) -> (0.8081, -1.5) projected
  line L55 (1.1513, -1.5) -> (0.8081, -1.5) projected
  line L56 (1.1513, -1.5) -> (1.4058, -1.5) projected
  line L57 (1.7121, -1.5) -> (1.4058, -1.5) projected
  line L58 (1.7121, -1.5) -> (2.057, -1.5) projected
  line L59 (2.057, -1.5) -> (2.2796, -1.5) projected
  line L60 (2.2796, -1.5) -> (2.9075, -1.5) projected
  line L61 (2.9075, -1.5) -> (3.2962, -1.5) projected
  line L62 (3.2962, -1.5) -> (4.9231, -1.5) projected
  line L63 (5.291, -1.5) -> (4.9231, -1.5) projected
  line L64 (5.291, -1.5) -> (5.5182, -1.5) projected
  line L65 (5.7302, -1.5) -> (5.5182, -1.5) projected
  line L66 (5.7302, -1.5) -> (5.1793, -1.5) projected
  line L67 (5.1793, -1.5) -> (5.2544, -1.5) projected
  line L68 (5.2544, -1.5) -> (5.7712, -1.5) projected
  line L69 (5.7712, -1.5) -> (6.1992, -1.5) projected
  line L70 (6.1992, -1.5) -> (8.3731, -1.5) projected
  line L71 (8.7161, -1.5) -> (8.3731, -1.5) projected
  line L72 (8.7161, -1.5) -> (8.8853, -1.5) projected
  line L73 (8.9744, -1.5) -> (8.8853, -1.5) projected
  line L74 (8.9744, -1.5) -> (7.602, -1.5) projected
  line L75 (7.602, -1.5) -> (7.5195, -1.5) projected
  line L76 (7.5195, -1.5) -> (7.8554, -1.5) projected
  line L77 (7.8554, -1.5) -> (8.265, -1.5) projected
  line L78 (8.265, -1.5) -> (10.6924, -1.5) projected
  line L79 (10.964, -1.5) -> (10.6924, -1.5) projected
  line L80 (10.964, -1.5) -> (11.0525, -1.5) projected
  line L81 (11.0066, -1.5) -> (11.0525, -1.5) projected
  line L82 (11.0066, -1.5) -> (8.9981, -1.5) projected
  line L83 (8.9981, -1.5) -> (8.769, -1.5) projected
  line L84 (8.769, -1.5) -> (8.8787, -1.5) projected
  line L85 (8.8787, -1.5) -> (9.2145, -1.5) projected
  line L86 (9.2145, -1.5) -> (11.5675, -1.5) projected
  line L87 (11.7312, -1.5) -> (11.5675, -1.5) projected
  line L88 (11.7312, -1.5) -> (11.7269, -1.5) projected
  line L89 (11.5523, -1.5) -> (11.7269, -1.5) projected
  line L90 (11.5523, -1.5) -> (9.1789, -1.5) projected
  line L91 (9.1789, -1.5) -> (8.8343, -1.5) projected
  line L92 (8.8343, -1.5) -> (8.7029, -1.5) projected
  line L93 (8.7029, -1.5) -> (8.9196, -1.5) projected
  line L94 (8.9196, -1.5) -> (10.8805, -1.5) projected
  line L95 (10.9141, -1.5) -> (10.8805, -1.5) projected
  line L96 (10.9141, -1.5) -> (10.8176, -1.5) projected
  line L97 (10.5377, -1.5) -> (10.8176, -1.5) projected
  line L98 (10.5377, -1.5) -> (8.12, -1.5) projected
  line L99 (8.12, -1.5) -> (7.7064, -1.5) projected
  line L100 (7.7064, -1.5) -> (7.3517, -1.5) projected
  line L101 (7.3517, -1.5) -> (7.4201, -1.5) projected
  line L102 (7.4201, -1.5) -> (8.7239, -1.5) projected
  line L103 (8.6229, -1.5) -> (8.7239, -1.5) projected
  line L104 (8.6229, -1.5) -> (8.4473, -1.5) projected
  line L105 (8.1, -1.5) -> (8.4473, -1.5) projected
  line L106 (8.1, -1.5) -> (5.9646, -1.5) projected
  line L107 (5.9646, -1.5) -> (5.5378, -1.5) projected
  line L108 (5.5378, -1.5) -> (5.0077, -1.5) projected
  line L109 (5.0077, -1.5) -> (4.9184, -1.5) projected
  line L110 (4.9184, -1.5) -> (5.3891, -1.5) projected
  line L111 (5.1671, -1.5) -> (5.3891, -1.5) projected
  line L112 (5.1671, -1.5) -> (4.9361, -1.5) projected
  line L113 (4.5684, -1.5) -> (4.9361, -1.5) projected
  line L114 (4.5684, -1.5) -> (3.0035, -1.5) projected
  line L115 (3.0035, -1.5) -> (2.6212, -1.5) projected
  line L116 (2.6212, -1.5) -> (1.9873, -1.5) projected
  line L117 (1.9873, -1.5) -> (1.7525, -1.5) projected
  line L118 (1.7525, -1.5) -> (1.3265, -1.5) projected
  line L119 (1.0136, -1.5) -> (1.3265, -1.5) projected
  line L120 (1.0136, -1.5) -> (0.7583, -1.5) projected
  line L121 (0.4197, -1.5) -> (0.7583, -1.5) projected
  line L122 (0.4197, -1.5) -> (-0.3632, -1.5) projected
  line L123 (-0.3632, -1.5) -> (-0.6494, -1.5) projected
  line L124 (-0.6494, -1.5) -> (-1.3015, -1.5) projected
  line L125 (-1.3015, -1.5) -> (-1.6502, -1.5) projected
  line L126 (-1.6502, -1.5) -> (-2.9152, -1.5) projected
  line L127 (-3.2769, -1.5) -> (-2.9152, -1.5) projected
  line L128 (-3.2769, -1.5) -> (-3.5219, -1.5) projected
  line L129 (-3.7856, -1.5) -> (-3.5219, -1.5) projected
  line L130 (-3.7856, -1.5) -> (-3.6808, -1.5) projected
  line L131 (-3.6808, -1.5) -> (-3.8323, -1.5) projected
  line L132 (-3.8323, -1.5) -> (-4.4145, -1.5) projected
  line L133 (-4.4145, -1.5) -> (-4.8299, -1.5) projected
  line L134 (-4.8299, -1.5) -> (-6.7633, -1.5) projected
  line L135 (-7.1248, -1.5) -> (-6.7633, -1.5) projected
  line L136 (-7.1248, -1.5) -> (-7.3265, -1.5) projected
  line L137 (-7.4797, -1.5) -> (-7.3265, -1.5) projected
  line L138 (-7.4797, -1.5) -> (-6.5013, -1.5) projected
  line L139 (-6.5013, -1.5) -> (-6.4976, -1.5) projected
  line L140 (-6.4976, -1.5) -> (-6.9313, -1.5) projected
  line L141 (-6.9313, -1.5) -> (-7.3574, -1.5) projected
  line L142 (-7.3574, -1.5) -> (-9.6979, -1.5) projected
  line L143 (-10.0105, -1.5) -> (-9.6979, -1.5) projected
  line L144 (-10.0105, -1.5) -> (-10.1416, -1.5) projected
  line L145 (-10.1636, -1.5) -> (-10.1416, -1.5) projected
  line L146 (-10.1636, -1.5) -> (-8.4438, -1.5) projected
  line L147 (-8.4438, -1.5) -> (-8.2853, -1.5) projected
  line L148 (-8.2853, -1.5) -> (-8.512, -1.5) projected
  line L149 (-8.512, -1.5) -> (-8.8911, -1.5) projected
  line L150 (-8.8911, -1.5) -> (-11.3228, -1.5) projected
  line L151 (-11.5442, -1.5) -> (-11.3228, -1.5) projected
  line L152 (-11.5442, -1.5) -> (-11.587, -1.5) projected
  line L153 (-11.4748, -1.5) -> (-11.587, -1.5) projected
  line L154 (-11.4748, -1.5) -> (-9.2459, -1.5) projected
  line L155 (-9.2459, -1.5) -> (-8.9541, -1.5) projected
  line L156 (-8.9541, -1.5) -> (-8.9431, -1.5) projected
  line L157 (-8.9431, -1.5) -> (-9.2241, -1.5) projected
  line L158 (-9.2241, -1.5) -> (-11.4184, -1.5) projected
  line L159 (-11.5188, -1.5) -> (-11.4184, -1.5) projected
  line L160 (-11.5188, -1.5) -> (-11.4675, -1.5) projected
  line L161 (-11.2363, -1.5) -> (-11.4675, -1.5) projected
  line L162 (-11.2363, -1.5) -> (-8.7993, -1.5) projected
  line L163 (-8.7993, -1.5) -> (-8.4136, -1.5) projected
  line L164 (-8.4136, -1.5) -> (-8.1664, -1.5) projected
  line L165 (-8.1664, -1.5) -> (-8.3114, -1.5) projected
  line L166 (-8.3114, -1.5) -> (-9.972, -1.5) projected
  line L167 (-9.9377, -1.5) -> (-9.972, -1.5) projected
  line L168 (-9.9377, -1.5) -> (-9.7993, -1.5) projected
  line L169 (-9.4803, -1.5) -> (-9.7993, -1.5) projected
  line L170 (-9.4803, -1.5) -> (-7.1643, -1.5) projected
  line L171 (-7.1643, -1.5) -> (-6.7368, -1.5) projected
  line L172 (-6.7368, -1.5) -> (-6.2867, -1.5) projected
  line L173 (-6.2867, -1.5) -> (-6.2761, -1.5) projected
  line L174 (-6.2761, -1.5) -> (-7.1788, -1.5) projected
  line L175 (-7.0145, -1.5) -> (-7.1788, -1.5) projected
  line L176 (-7.0145, -1.5) -> (-6.8076, -1.5) projected
  line L177 (-6.4439, -1.5) -> (-6.8076, -1.5) projected
  line L178 (-6.4439, -1.5) -> (-4.5617, -1.5) projected
  line L179 (-4.5617, -1.5) -> (-4.1501, -1.5) projected
  line L180 (-4.1501, -1.5) -> (-3.5581, -1.5) projected
  line L181 (-3.5581, -1.5) -> (-3.3932, -1.5) projected
  line L182 (-3.3932, -1.5) -> (-3.416, -1.5) projected
  line L183 (-3.1439, -1.5) -> (-3.416, -1.5) projected
  line L184 (-3.1439, -1.5) -> (-2.8965, -1.5) projected
  line L185 (-2.5373, -1.5) -> (-2.8965, -1.5) projected
  line L186 (-2.5373, -1.5) -> (-1.343, -1.5) projected
  line L187 (-1.343, -1.5) -> (-1.003, -1.5) projected
  line L188 (-1.003, -1.5) -> (-0.3488, -1.5) projected
  line L189 (-3.9904, 1.5) -> (-3.9904, 1.5) projected
  line L190 (-3.9904, -1.5) -> (-3.9904, 1.5) projected
  line L191 (-3.9904, -1.5) -> (-3.9904, -1.5) projected
  line L192 (-3.9904, -1.5) -> (-3.9904, 1.5) projected
  line L193 (-5.1, -1.5) -> (-3.9904, -0.3904)
  line L194 (-3.9904, -1.5) -> (-3.9904, 1.5) projected
  line L195 (-3.9904, -0.3904) -> (-3.9904, -1.5)
  line L196 (-3.9904, -1.5) -> (-5.1, -1.5)
  line L197 (-16.2574, 0) -> (16.3961, 0) projected
  line L198 (-4.5218, 1.5) -> (-4.5218, -1.5)
  line L199 (-4.8652, 1.5) -> (-4.5218, 1.5)
  line L200 (-4.8652, 1.5) -> (-4.8652, -1.5)
  line L201 (-3.0178, 1.5) -> (-4.4008, 1.5)
  line L202 (-4.4008, 1.5) -> (-4.5218, 1.5)
  line L203 (-4.5218, 1.5) -> (-4.8652, 1.5)
  line L204 (-4.8652, 1.5) -> (-4.8395, 1.5)
  line L205 (-4.8395, 1.5) -> (-3.9904, 1.5)
  line L206 (-3.9904, 1.5) -> (-4.8395, 1.5)
  line L207 (-4.8395, 1.5) -> (-4.8652, 1.5)
  line L208 (-4.8652, 1.5) -> (-4.5218, 1.5)
  line L209 (-4.5218, 1.5) -> (-4.4008, 1.5)
  line L210 (-4.4008, 1.5) -> (-3.0178, 1.5)
  line L211 (-3.7856, 1.5) -> (-3.5219, 1.5)
  line L212 (-3.7856, 1.5) -> (-3.6808, 1.5)
  line L213 (-3.6808, 1.5) -> (-3.8323, 1.5)
  line L214 (-3.8323, 1.5) -> (-4.4145, 1.5)
  line L215 (-4.4145, 1.5) -> (-4.8299, 1.5)
  line L216 (-4.8299, 1.5) -> (-6.7633, 1.5)
  line L217 (-6.4439, 1.5) -> (-4.5617, 1.5)
  line L218 (-4.5617, 1.5) -> (-4.1501, 1.5)
  line L219 (-4.1501, 1.5) -> (-3.5581, 1.5)
  line L220 (-3.9904, 1.5) -> (-3.9904, -1.5)
  line L221 (-3.9904, 1.5) -> (-3.9904, -1.5)
  line L222 (-5.1, 1.5) -> (-3.9904, 0.3904)
  line L223 (-3.9904, 1.5) -> (-3.9904, -1.5)
  line L224 (-3.9904, 0.3904) -> (-3.9904, 1.5)
  line L225 (-3.9904, 1.5) -> (-5.1, 1.5)
  point P0 (0, 0)
  dimension "d85" = 45
  dimension "d86" = 5.1
  constraints: 62 end point, 33 symmetric about line, 4 point on line, 2 collinear
  measures "d85" angle of L196 L193
  measures "d86" distance from line of L4 L193.start
revolve "Revolution1" cut sketch "Sketch6" angle 360 about axis through (0, 0, 0) along (0, -1, 0) contours L1 L222 L3 L0 | L202 L201 L190 L222 L1 | L222 L216 L3 | L193 L190 L40 L41 L1 | L1 L2 L3 L193 | L3 L134 L193
equation "\"d23\" = G_pitch_diam"
equation "\"d25\" = G_dedendum"
equation "\"d26\" = G_addendum"
equation "\"d27\" = G_pressure_ang"
equation "\"d28\" = 2 * G_base_circ"
equation "\"d29\" = G_pressure_ang"
equation "\"d30\" = G_clearance"
equation "\"d31\" = 2 * G_fillet_r"
equation "\"d32\" = 0.5 * G_thickness_tooth"
equation "\"d36\" = H_tip_circ_diam_shaft"
equation "\"d37\" = H_root_circ_diam_shaft"
equation "\"d38\" = H_pressure_ang"
equation "\"d39\" = H_base_form_circ_diam_shaft"
equation "\"d40\" = H_dedendum"
equation "\"d41\" = 0.5 * H_pitch"
equation "\"d42\" = 2 * H_root_fillet_r"
equation "\"d58\" = H_tip_circ_diam_hub"
equation "\"d59\" = 2 * H_addendum + H_tip_circ_diam_hub + 2 * H_dedendum"
equation "\"d60\" = H_tip_circ_diam_hub + 2 * H_addendum"
equation "\"d61\" = 0.5 * H_pitch"
equation "\"G_pitch_diam\" = 21"
equation "\"G_clearance\" = G_dedendum - G_addendum"
equation "\"G_addendum\" = G_module"
equation "\"G_dedendum\" = 1.25 * G_module"
equation "\"G_fillet_r\" = G_clearance"
equation "\"G_thickness_tooth\" = 0.5 * G_pitch_circ"
equation "\"G_pitch_circ\" = 3.1416 * G_module"
equation "\"G_pressure_ang\" = 20deg"
equation "\"H_pressure_ang\" = 30deg"
equation "\"H_dedendum\" = 0.65 * H_module"
equation "\"H_pitch\" = 3.1416 * H_module"
equation "\"H_root_fillet_r\" = 0.16 * H_module"
equation "\"H_module\" = 1"
equation "\"H_addendum_mod_shaft\" = 0.45"
equation "\"H_addendum_mod_hub\" = -H_addendum_mod_shaft"
equation "\"H_addendum\" = 0.45 * H_module"
equation "\"G_base_circ\" = 9.866773"
equation "\"H_tip_circ_diam_shaft\" = 9.8"
equation "\"H_root_circ_diam_shaft\" = 7.6"
equation "\"H_base_form_circ_diam_shaft\" = 7.5"
equation "\"H_tip_circ_diam_hub\" = 8"
equation "\"G_module\" = 1.235294"
body "Solid1"
